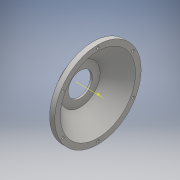
# Autodesk Inventor part: Деталь 6
Saved by Autodesk Inventor 2016 SP1 (Build 200210100, 210)
## iProperties
Created: 2016-05-02
Part Number: Деталь 6
Material: Типовые
Document SubType Name: Modeling
Designer: AS
Density: 1 g/cm^3
Appearance: По умолчанию
Mass: 244.158 g
Surface Area: 696.966 cm^2
Volume: 244.158 cm^3
Author: AS
Autodesk Inventor part; units mm, degrees
ref_plane "YZ Plane" through (0, 0, 0) normal (1, 0, 0) x (0, 1, 0)
ref_plane "XZ Plane" through (0, 0, 0) normal (0, 1, 0) x (-1, 0, 0)
ref_plane "XY Plane" through (0, 0, 0) normal (0, 0, 1) x (1, 0, 0)
sketch "Эскиз1" plane through (0, 0, 0) normal (0, 0, 1) x (1, 0, 0)
  line L0 (0, 81) -> (0, 93)
  line L1 (0, 93) -> (-11, 93)
  line L2 (-11, 93) -> (-11, 81.2677)
  line L3 (-11, 81.2677) -> (-42, 50)
  line L4 (-42, 50) -> (-42, 26)
  line L5 (-42, 26) -> (-38, 26)
  line L6 (-38, 26) -> (-38, 42.6719)
  line L7 (-38, 42.6719) -> (0, 81)
  line L8 (0, 0) -> (0, 108.7974) construction
  line L9 (-50.4, 0) -> (8.4, 0) projected
  dimension "d0" = 11
  dimension "d1" = 12
  dimension "d2" = 24
  dimension "d3" = 4
  dimension "d4" = 8
  dimension "d5" = 67
  dimension "d6" = 42
  dimension "d7" = 93
  constraints: 18 end point, 4 perpendicular, 2 parallel, 2 vertical, 1 point on line
  measures "d0" distance between parallel lines of L2 L0
  measures "d1" distance of L0.start L0.end
  measures "d2" distance of L3.end L4.end
  measures "d3" distance of L4.end L5.end
  measures "d4" distance between parallel lines of L3 L7
  measures "d5" vertical distance of L4.end L1.end
  measures "d6" distance between parallel lines of L4 L0
  measures "d7" distance from line of L8.start L1
revolve "Вращение1" add sketch "Эскиз1" angle 360 about axis through (-10, 0, 0) along (1, 0, 0)
hole "Отверстие1" at (-11, -0.0233, 87.0155) direction (1, 0, 0) diameter 5 end through all counterbore diameter 9 counterbore depth 5
pattern_circular "Круговой массив1" count 6 over 360 about axis through (-10, 0, 0) along (1, 0, 0) of "Отверстие1"
